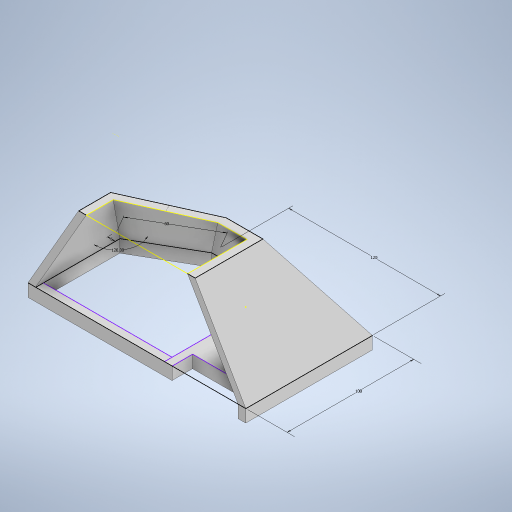
# Autodesk Inventor part: Part2
Saved by Autodesk Inventor 2023 (Build 270158000, 158)
## iProperties
Created: 2022-06-24
Part Number: Part2
Material: Generic
Document SubType Name: Modeling
Designer: Dan
Density: 1 g/cm^3
Appearance: Default
Author: Dan
Autodesk Inventor part; units mm, degrees
ref_plane "YZ Plane" through (0, 0, 0) normal (1, 0, 0) x (0, 1, 0)
ref_plane "XZ Plane" through (0, 0, 0) normal (0, 1, 0) x (-1, 0, 0)
sketch "Base Sketch" plane through (0, 0, 0) normal (0, 1, 0) x (-1, 0, 0)
  line L0 (0, 0) -> (0, -100)
  line L1 (0, -100) -> (120, -100)
  line L2 (120, -100) -> (171.961524, -70)
  line L3 (171.961524, -70) -> (171.961524, 0)
  line L4 (171.961524, 0) -> (0, 0)
  line L5 (165.961524, 0) -> (165.961524, -66.535898)
  line L6 (165.961524, -66.535898) -> (120, -93.071797)
  line L7 (142.980762, -79.803848) -> (145.980762, -85) construction
  line L8 (165.961524, -66.535898) -> (171.961524, -66.535898) construction
  line L9 (120, -93.071797) -> (6, -93.071797)
  line L10 (6, -93.071797) -> (6, 0)
  line L11 (6, -93.071797) -> (0, -93.071797) construction
  line L12 (120, -93.071797) -> (6, -93.071797)
  line L13 (6, -93.071797) -> (6, -50.829914)
  line L14 (64.279786, -42.471598) -> (64.279786, 0)
  line L15 (64.279786, -42.471598) -> (79.982467, -50.95258)
  line L16 (79.982467, -50.95258) -> (79.982467, -93.071797)
  line L17 (73.630775, -93.071797) -> (73.630775, -56.839275)
  line L18 (73.630775, -56.839275) -> (64.279786, -51.788827)
  line L19 (64.279786, -51.788827) -> (6, -51.788827)
  line L20 (15.591156, -23.128064) -> (15.591156, -42.842523)
  line L21 (15.591156, -42.842523) -> (6, -46.535898)
  line L22 (165.961524, -5.975934) -> (64.279786, -5.975934)
  line L23 (58.217157, 0) -> (58.217157, -16.174978)
  line L24 (58.217157, -16.174978) -> (15.591156, -16.174978)
  line L25 (15.591156, -23.128064) -> (6, -17.935692)
  line L26 (15.591156, -16.174978) -> (6, -10.994816)
  dimension "d0" = 100
  dimension "d1" = 120
  dimension "d3" = 60
  dimension "d4" = 120
  dimension "d5" = 6
  constraints: 54 end point, 16 point on line, 11 perpendicular, 5 vertical, 3 horizontal, 3 midpoint, 3 parallel, 2 equal length
  measures "d0" distance of L0.start L0.end
  measures "d1" angle of L2 L3
  measures "d3" distance of L1.end L2.end
  measures "d4" distance of L0.end L1.end
  measures "d5" distance of L5.end L8.end
sketch3d "3D Scaffold Sketch"
ref_plane "Ceiling" through (-46, 69.282032, -46.883775) normal (0, 1, 0) x (0, 0, 1)
sketch "Ceiling Sketch" plane through (-46, 69.282032, -46.883775) normal (0, 1, 0) x (0, 0, 1)
  line L0 (46.883775, -79.961524) -> (46.883775, 0)
  line L1 (0, 0) -> (46.883775, 0)
  line L2 (0, -22.962669) -> (0, 0)
  line L3 (0, -22.962669) -> (25.614297, -79.961524)
  line L4 (46.883775, -79.961524) -> (25.614297, -79.961524)
  line L5 (46.883775, 0) -> (46.883775, 6)
  line L6 (46.883775, 6) -> (-6.577994, 6)
  line L7 (-6.577994, 6) -> (-6.577994, -22.962669)
  line L8 (-6.577994, -22.962669) -> (21.732598, -85.961524)
  line L9 (21.732598, -85.961524) -> (46.883775, -85.961524)
  line L10 (46.883775, -85.961524) -> (46.883775, -79.961524)
  line L11 (-19.652123, -119.961524) -> (-19.652123, -125.961524) construction
  line L12 (12.807148, -51.462096) -> (7.334356, -53.921474) construction
  point P0 (46.883775, 46)
  constraints: 14 end point, 4 perpendicular, 3 equal length, 2 parallel, 2 point on line, 1 horizontal alignment, 1 midpoint, 1 vertical
sketch3d "3D Scaffold Finish Sketch"
sketch "Base Sketch outline for Loft1" plane through (0, 0, 0) normal (0, 1, 0) x (-1, 0, 0)
  line L0 (6, 0) -> (0, 0)
  line L1 (6, -93.071797) -> (6, 0)
  line L2 (120, -93.071797) -> (6, -93.071797)
  line L3 (165.961524, -66.535898) -> (120, -93.071797)
  line L4 (165.961524, 0) -> (165.961524, -66.535898)
  line L5 (171.961524, 0) -> (165.961524, 0)
  line L6 (171.961524, -70) -> (171.961524, 0)
  line L7 (120, -100) -> (171.961524, -70)
  line L8 (0, -100) -> (120, -100)
  line L9 (0, 0) -> (0, -100)
sketch "Ceiling Sketch outline for Loft1" plane through (-46, 69.282032, -46.883775) normal (0, 1, 0) x (0, 0, 1)
  line L0 (46.883775, -85.961524) -> (46.883775, -79.961524)
  line L1 (21.732598, -85.961524) -> (46.883775, -85.961524)
  line L2 (-6.577994, -22.962669) -> (21.732598, -85.961524)
  line L3 (-6.577994, 6) -> (-6.577994, -22.962669)
  line L4 (46.883775, 6) -> (-6.577994, 6)
  line L5 (46.883775, 0) -> (46.883775, 6)
  line L6 (0, 0) -> (46.883775, 0)
  line L7 (0, -22.962669) -> (0, 0)
  line L8 (25.614297, -79.961524) -> (0, -22.962669)
  line L9 (46.883775, -79.961524) -> (25.614297, -79.961524)
loft "Loft1" add profiles "Base Sketch outline for Loft1", "Ceiling Sketch outline for Loft1"
extrude "Base Extrusion" add sketch "Base Sketch" against normal blind 10 separate body contours L4 L10 L9 L6 L5 L3 L2 L1 L0 | L4 L14 L15 L16 L9 L17 L18 L19 L10 L21 L20 L25 L26 L24 L23 | L4 L5 L22 L14
sketch "Sketch4" plane through (0, -10, 0) normal (0, -1, 0) x (1, 0, 0)
  line L0 (-47.583857, -30.738827) -> (-31.583857, -30.738827) construction
  line L1 (-31.583857, -30.738827) -> (-31.583857, -44.838827) construction
  line L2 (-31.583857, -44.838827) -> (-47.583857, -44.838827) construction
  line L3 (-47.583857, -44.838827) -> (-47.583857, -30.738827) construction
  line L4 (-39.583857, -44.838827) -> (-39.583857, -30.738827) construction
  line L5 (-47.583857, -37.788827) -> (-31.583857, -37.788827) construction
  line L6 (-64.279786, -51.788827) -> (-6, -51.788827)
  point P0 (0, 0)
  dimension "d42" = 14.1
  dimension "d43" = 16
  dimension "d45" = 14
  constraints: 12 end point, 4 coincident, 4 midpoint, 2 parallel, 1 horizontal, 1 perpendicular
  measures "d42" distance of L2.end L0.start
  measures "d43" distance of L1.end L2.end
  measures "d45" distance between parallel lines of L6 L5
hole "Hole1" at (-47.583857, -10, -30.738827) at (-47.583857, -10, -44.838827) at (-31.583857, -10, -30.738827) at (-31.583857, -10, -44.838827) direction (0, 1, 0) diameter 3.4 end through all counterbore diameter 6.5 counterbore depth 3.4 bodies 2 clearance for "Socket Head Cap Screw ISO 4762" size "M3" standard "ISO"
body "Solid1"
body "Solid3"
